Autodesk Fusion 360 part; units mm, degrees
note: some values were not read from the file. Set by a fixed rule: which sketch regions a step uses.
(part 8 of 59)
  spline S40 degree 5 poles (-13.0527, 40.6181) (-13.0525, 40.6154) (-13.0521, 40.61) (-13.0515, 40.6019) (-13.0506, 40.5911) (-13.0495, 40.5777) (-13.0484, 40.5644) (-13.0473, 40.551) (-13.0462, 40.5377) (-13.0451, 40.5244) (-13.0439, 40.5112) (-13.0427, 40.4979) (-13.0415, 40.4848) (-13.0404, 40.4716) (-13.0391, 40.4585) (-13.0379, 40.4454) (-13.0367, 40.4323) (-13.0354, 40.4193) (-13.0342, 40.4063) (-13.0329, 40.3934) (-13.0316, 40.3805) (-13.0303, 40.3676) (-13.029, 40.3547) (-13.0276, 40.3419) (-13.0263, 40.3291) (-13.0249, 40.3164) (-13.0236, 40.3037) (-13.0222, 40.291) (-13.0208, 40.2784) (-13.0194, 40.2658) (-13.018, 40.2532) (-13.0165, 40.2406) (-13.0151, 40.2281) (-13.0136, 40.2157) (-13.0122, 40.2032) (-13.0107, 40.1908) (-13.0092, 40.1785) (-13.0077, 40.1661) (-13.0062, 40.1539) (-13.0047, 40.1416) (-13.0031, 40.1294) (-13.0016, 40.1172) (-13, 40.105) (-12.9984, 40.0929) (-12.9968, 40.0809) (-12.9952, 40.0688) (-12.9936, 40.0568) (-12.992, 40.0449) (-12.9904, 40.0329) (-12.9887, 40.021) (-12.9871, 40.0092) (-12.9854, 39.9974) (-12.9838, 39.9856) (-12.9821, 39.9738) (-12.9804, 39.9621) (-12.9787, 39.9505) (-12.977, 39.9388) (-12.9752, 39.9273) (-12.9735, 39.9157) (-12.9718, 39.9042) (-12.97, 39.8927) (-12.9682, 39.8813) (-12.9665, 39.8699) (-12.9647, 39.8585) (-12.9629, 39.8472) (-12.9611, 39.8359) (-12.9593, 39.8247) (-12.9574, 39.8135) (-12.9556, 39.8023) (-12.9538, 39.7912) (-12.9519, 39.7801) (-12.9501, 39.7691) (-12.9482, 39.7581) (-12.9463, 39.7471) (-12.9445, 39.7362) (-12.9426, 39.7253) (-12.9407, 39.7145) (-12.9388, 39.7037) (-12.9368, 39.6929) (-12.9349, 39.6822) (-12.933, 39.6715) (-12.9311, 39.6609) (-12.9291, 39.6503) (-12.9272, 39.6397) (-12.9252, 39.6292) (-12.9232, 39.6188) (-12.9213, 39.6083) (-12.9193, 39.5979) (-12.9173, 39.5876) (-12.9153, 39.5773) (-12.9133, 39.5671) (-12.9113, 39.5568) (-12.9093, 39.5467) (-12.9072, 39.5365) (-12.9052, 39.5265) (-12.9032, 39.5164) (-12.9011, 39.5064) (-12.8991, 39.4965) (-12.8971, 39.4866) (-12.895, 39.4767) (-12.8929, 39.4669) (-12.8909, 39.4571) (-12.8888, 39.4474) (-12.8867, 39.4377) (-12.8847, 39.4281) (-12.8826, 39.4185) (-12.8805, 39.4089) (-12.8784, 39.3994) (-12.8763, 39.39) (-12.8742, 39.3806) (-12.8721, 39.3712) (-12.87, 39.3619) (-12.8679, 39.3526) (-12.8658, 39.3434) (-12.8636, 39.3342) (-12.8615, 39.3251) (-12.8594, 39.316) (-12.8573, 39.3069) (-12.8551, 39.298) (-12.853, 39.289) (-12.8509, 39.2801) (-12.8487, 39.2713) (-12.8466, 39.2625) (-12.8445, 39.2537) (-12.8423, 39.2451) (-12.8402, 39.2364) (-12.838, 39.2278) (-12.8359, 39.2193) (-12.8337, 39.2108) (-12.8316, 39.2023) (-12.8294, 39.1939) (-12.8273, 39.1856) (-12.8251, 39.1773) (-12.823, 39.169) (-12.8208, 39.1608) (-12.8187, 39.1527) (-12.8166, 39.1446) (-12.8144, 39.1365) (-12.8123, 39.1286) (-12.8101, 39.1206) (-12.808, 39.1127) (-12.8058, 39.1049) (-12.8037, 39.0971) (-12.8016, 39.0894) (-12.7994, 39.0817) (-12.7973, 39.0741) (-12.7952, 39.0665) (-12.793, 39.059) (-12.7909, 39.0516) (-12.7888, 39.0442) (-12.7867, 39.0368) (-12.7845, 39.0296) (-12.7824, 39.0223) (-12.7803, 39.0151) (-12.7782, 39.008) (-12.7761, 39.0009) (-12.774, 38.9939) (-12.772, 38.987) (-12.7699, 38.9801) (-12.7678, 38.9733) (-12.7657, 38.9665) (-12.7637, 38.9598) (-12.7616, 38.9531) (-12.7596, 38.9465) (-12.7575, 38.9399) (-12.7555, 38.9335) (-12.7534, 38.927) (-12.7514, 38.9207) (-12.7494, 38.9144) (-12.7474, 38.9081) (-12.7454, 38.9019) (-12.7434, 38.8958) (-12.7414, 38.8897) (-12.7395, 38.8837) (-12.7375, 38.8778) (-12.7356, 38.8719) (-12.7336, 38.8661) (-12.7317, 38.8604) (-12.7298, 38.8547) (-12.7279, 38.8491) (-12.726, 38.8435) (-12.7241, 38.838) (-12.7222, 38.8326) (-12.7204, 38.8273) (-12.7185, 38.822) (-12.7167, 38.8167) (-12.7149, 38.8116) (-12.7131, 38.8065) (-12.7113, 38.8015) (-12.7095, 38.7965) (-12.7077, 38.7916) (-12.706, 38.7868) (-12.7043, 38.782) (-12.7026, 38.7774) (-12.7009, 38.7728) (-12.6992, 38.7682) (-12.6975, 38.7638) (-12.6959, 38.7594) (-12.6943, 38.755) (-12.6927, 38.7508) (-12.6911, 38.7466) (-12.6895, 38.7425) (-12.688, 38.7385) (-12.6864, 38.7345) (-12.6849, 38.7307) (-12.6834, 38.7269) (-12.682, 38.7231) (-12.6806, 38.7195) (-12.6791, 38.7159) (-12.6778, 38.7124) (-12.6764, 38.709) (-12.675, 38.7057) (-12.6737, 38.7024) (-12.6724, 38.6993) (-12.6712, 38.6962) (-12.6699, 38.6932) (-12.6687, 38.6903) (-12.6676, 38.6874) (-12.6664, 38.6847) (-12.6653, 38.682) (-12.6642, 38.6794) (-12.6631, 38.6769) (-12.6621, 38.6745) (-12.6611, 38.6722) (-12.6602, 38.67) (-12.6592, 38.6678) (-12.6583, 38.6658) (-12.6575, 38.6638) (-12.6567, 38.6619) (-12.6559, 38.6602) (-12.6551, 38.6585) (-12.6544, 38.6569) (-12.6538, 38.6554) (-12.6531, 38.654) (-12.6526, 38.6527) (-12.652, 38.6515) (-12.6515, 38.6504) (-12.651, 38.6495) (-12.6506, 38.6486) (-12.6503, 38.6478) (-12.65, 38.6471) (-12.6497, 38.6467) (-12.6496, 38.6464) (-12.6495, 38.6462) (-12.6495, 38.6461) knots -1 -1 -1 -1 -1 -1 -0.99583333 -0.99166667 -0.9875 -0.98333333 -0.97916667 -0.975 -0.97083333 -0.96666667 -0.9625 -0.95833333 -0.95416667 -0.95 -0.94583333 -0.94166667 -0.9375 -0.93333333 -0.92916667 -0.925 -0.92083333 -0.91666667 -0.9125 -0.90833333 -0.90416667 -0.9 -0.89583333 -0.89166667 -0.8875 -0.88333333 -0.87916667 -0.875 -0.87083333 -0.86666667 -0.8625 -0.85833333 -0.85416667 -0.85 -0.84583333 -0.84166667 -0.8375 -0.83333333 -0.82916667 -0.825 -0.82083333 -0.81666667 -0.8125 -0.80833333 -0.80416667 -0.8 -0.79583333 -0.79166667 -0.7875 -0.78333333 -0.77916667 -0.775 -0.77083333 -0.76666667 -0.7625 -0.75833333 -0.75416667 -0.75 -0.74583333 -0.74166667 -0.7375 -0.73333333 -0.72916667 -0.725 -0.72083333 -0.71666667 -0.7125 -0.70833333 -0.70416667 -0.7 -0.69583333 -0.69166667 -0.6875 -0.68333333 -0.67916667 -0.675 -0.67083333 -0.66666667 -0.6625 -0.65833333 -0.65416667 -0.65 -0.64583333 -0.64166667 -0.6375 -0.63333333 -0.62916667 -0.625 -0.62083333 -0.61666667 -0.6125 -0.60833333 -0.60416667 -0.6 -0.59583333 -0.59166667 -0.5875 -0.58333333 -0.57916667 -0.575 -0.57083333 -0.56666667 -0.5625 -0.55833333 -0.55416667 -0.55 -0.54583333 -0.54166667 -0.5375 -0.53333333 -0.52916667 -0.525 -0.52083333 -0.51666667 -0.5125 -0.50833333 -0.50416667 -0.5 -0.49583333 -0.49166667 -0.4875 -0.48333333 -0.47916667 -0.475 -0.47083333 -0.46666667 -0.4625 -0.45833333 -0.45416667 -0.45 -0.44583333 -0.44166667 -0.4375 -0.43333333 -0.42916667 -0.425 -0.42083333 -0.41666667 -0.4125 -0.40833333 -0.40416667 -0.4 -0.39583333 -0.39166667 -0.3875 -0.38333333 -0.37916667 -0.375 -0.37083333 -0.36666667 -0.3625 -0.35833333 -0.35416667 -0.35 -0.34583333 -0.34166667 -0.3375 -0.33333333 -0.32916667 -0.325 -0.32083333 -0.31666667 -0.3125 -0.30833333 -0.30416667 -0.3 -0.29583333 -0.29166667 -0.2875 -0.28333333 -0.27916667 -0.275 -0.27083333 -0.26666667 -0.2625 -0.25833333 -0.25416667 -0.25 -0.24583333 -0.24166667 -0.2375 -0.23333333 -0.22916667 -0.225 -0.22083333 -0.21666667 -0.2125 -0.20833333 -0.20416667 -0.2 -0.19583333 -0.19166667 -0.1875 -0.18333333 -0.17916667 -0.175 -0.17083333 -0.16666667 -0.1625 -0.15833333 -0.15416667 -0.15 -0.14583333 -0.14166667 -0.1375 -0.13333333 -0.12916667 -0.125 -0.12083333 -0.11666667 -0.1125 -0.10833333 -0.10416667 -0.1 -0.09583333 -0.09166667 -0.0875 -0.08333333 -0.07916667 -0.075 -0.07083333 -0.06666667 -0.0625 -0.05833333 -0.05416667 -0.05 -0.04583333 -0.04166667 -0.0375 -0.03333333 -0.02916667 -0.025 -0.02083333 -0.01666667 -0.0125 -0.00833333 -0.00416667 0 0 0 0 0 0
  spline S41 degree 5 poles (-20.3781, -10.8609) (-20.3757, -10.8596) (-20.371, -10.8571) (-20.3639, -10.8532) (-20.3544, -10.848) (-20.3426, -10.8416) (-20.3308, -10.8351) (-20.319, -10.8287) (-20.3073, -10.8222) (-20.2957, -10.8158) (-20.284, -10.8094) (-20.2724, -10.8029) (-20.2609, -10.7965) (-20.2493, -10.79) (-20.2379, -10.7836) (-20.2264, -10.7771) (-20.215, -10.7707) (-20.2036, -10.7643) (-20.1922, -10.7578) (-20.1809, -10.7514) (-20.1697, -10.745) (-20.1584, -10.7385) (-20.1472, -10.7321) (-20.136, -10.7257) (-20.1249, -10.7193) (-20.1138, -10.7128) (-20.1028, -10.7064) (-20.0917, -10.7) (-20.0808, -10.6936) (-20.0698, -10.6872) (-20.0589, -10.6807) (-20.048, -10.6743) (-20.0372, -10.6679) (-20.0264, -10.6615) (-20.0156, -10.6551) (-20.0049, -10.6487) (-19.9942, -10.6423) (-19.9836, -10.636) (-19.973, -10.6296) (-19.9624, -10.6232) (-19.9518, -10.6168) (-19.9413, -10.6104) (-19.9309, -10.6041) (-19.9205, -10.5977) (-19.9101, -10.5914) (-19.8997, -10.585) (-19.8894, -10.5786) (-19.8791, -10.5723) (-19.8689, -10.566) (-19.8587, -10.5596) (-19.8486, -10.5533) (-19.8384, -10.547) (-19.8284, -10.5406) (-19.8183, -10.5343) (-19.8083, -10.528) (-19.7984, -10.5217) (-19.7884, -10.5154) (-19.7785, -10.5091) (-19.7687, -10.5029) (-19.7589, -10.4966) (-19.7491, -10.4903) (-19.7394, -10.484) (-19.7297, -10.4778) (-19.72, -10.4715) (-19.7104, -10.4653) (-19.7009, -10.4591) (-19.6913, -10.4528) (-19.6818, -10.4466) (-19.6724, -10.4404) (-19.663, -10.4342) (-19.6536, -10.428) (-19.6443, -10.4218) (-19.635, -10.4156) (-19.6257, -10.4095) (-19.6165, -10.4033) (-19.6073, -10.3971) (-19.5982, -10.391) (-19.5891, -10.3849) (-19.5801, -10.3787) (-19.5711, -10.3726) (-19.5621, -10.3665) (-19.5532, -10.3604) (-19.5443, -10.3543) (-19.5354, -10.3483) (-19.5266, -10.3422) (-19.5179, -10.3361) (-19.5091, -10.3301) (-19.5005, -10.3241) (-19.4918, -10.318) (-19.4832, -10.312) (-19.4747, -10.306) (-19.4662, -10.3) (-19.4577, -10.2941) (-19.4493, -10.2881) (-19.4409, -10.2822) (-19.4325, -10.2762) (-19.4242, -10.2703) (-19.416, -10.2644) (-19.4078, -10.2585) (-19.3996, -10.2526) (-19.3914, -10.2467) (-19.3834, -10.2408) (-19.3753, -10.235) (-19.3673, -10.2292) (-19.3593, -10.2233) (-19.3514, -10.2175) (-19.3436, -10.2118) (-19.3357, -10.206) (-19.3279, -10.2002) (-19.3202, -10.1945) (-19.3125, -10.1887) (-19.3048, -10.183) (-19.2972, -10.1773) (-19.2897, -10.1716) (-19.2821, -10.166) (-19.2747, -10.1603) (-19.2672, -10.1547) (-19.2598, -10.1491) (-19.2525, -10.1435) (-19.2452, -10.1379) (-19.2379, -10.1323) (-19.2307, -10.1268) (-19.2236, -10.1212) (-19.2165, -10.1157) (-19.2094, -10.1102) (-19.2024, -10.1048) (-19.1954, -10.0993) (-19.1884, -10.0939) (-19.1815, -10.0884) (-19.1747, -10.083) (-19.1679, -10.0777) (-19.1611, -10.0723) (-19.1544, -10.067) (-19.1478, -10.0617) (-19.1412, -10.0564) (-19.1346, -10.0511) (-19.1281, -10.0458) (-19.1216, -10.0406) (-19.1152, -10.0354) (-19.1088, -10.0302) (-19.1025, -10.025) (-19.0962, -10.0199) (-19.09, -10.0148) (-19.0838, -10.0097) (-19.0776, -10.0046) (-19.0715, -9.9996) (-19.0655, -9.9945) (-19.0595, -9.9895) (-19.0536, -9.9846) (-19.0477, -9.9796) (-19.0418, -9.9747) (-19.036, -9.9698) (-19.0303, -9.9649) (-19.0246, -9.9601) (-19.0189, -9.9553) (-19.0133, -9.9505) (-19.0077, -9.9457) (-19.0022, -9.941) (-18.9968, -9.9363) (-18.9914, -9.9316) (-18.986, -9.927) (-18.9807, -9.9223) (-18.9755, -9.9177) (-18.9703, -9.9132) (-18.9651, -9.9087) (-18.96, -9.9042) (-18.955, -9.8997) (-18.95, -9.8953) (-18.9451, -9.8909) (-18.9402, -9.8865) (-18.9353, -9.8821) (-18.9306, -9.8778) (-18.9258, -9.8736) (-18.9211, -9.8693) (-18.9165, -9.8651) (-18.9119, -9.8609) (-18.9074, -9.8568) (-18.903, -9.8527) (-18.8986, -9.8486) (-18.8942, -9.8446) (-18.8899, -9.8406) (-18.8856, -9.8367) (-18.8814, -9.8328) (-18.8773, -9.8289) (-18.8732, -9.825) (-18.8692, -9.8212) (-18.8652, -9.8175) (-18.8613, -9.8138) (-18.8574, -9.8101) (-18.8536, -9.8065) (-18.8499, -9.8029) (-18.8462, -9.7993) (-18.8426, -9.7958) (-18.839, -9.7923) (-18.8355, -9.7889) (-18.832, -9.7855) (-18.8286, -9.7822) (-18.8252, -9.7789) (-18.822, -9.7757) (-18.8187, -9.7725) (-18.8156, -9.7693) (-18.8124, -9.7662) (-18.8094, -9.7632) (-18.8064, -9.7602) (-18.8035, -9.7572) (-18.8006, -9.7543) (-18.7978, -9.7515) (-18.7951, -9.7487) (-18.7924, -9.7459) (-18.7897, -9.7433) (-18.7872, -9.7406) (-18.7847, -9.738) (-18.7823, -9.7355) (-18.7799, -9.7331) (-18.7776, -9.7307) (-18.7753, -9.7283) (-18.7732, -9.726) (-18.771, -9.7238) (-18.769, -9.7216) (-18.767, -9.7195) (-18.7651, -9.7175) (-18.7632, -9.7155) (-18.7615, -9.7136) (-18.7597, -9.7117) (-18.7581, -9.7099) (-18.7565, -9.7082) (-18.755, -9.7066) (-18.7536, -9.705) (-18.7522, -9.7035) (-18.7509, -9.702) (-18.7497, -9.7007) (-18.7485, -9.6994) (-18.7474, -9.6982) (-18.7464, -9.697) (-18.7455, -9.696) (-18.7446, -9.695) (-18.7438, -9.6941) (-18.7431, -9.6933) (-18.7424, -9.6925) (-18.7419, -9.6919) (-18.7414, -9.6913) (-18.741, -9.6909) (-18.7408, -9.6907) (-18.7407, -9.6905) (-18.7406, -9.6904) knots -1 -1 -1 -1 -1 -1 -0.99583333 -0.99166667 -0.9875 -0.98333333 -0.97916667 -0.975 -0.97083333 -0.96666667 -0.9625 -0.95833333 -0.95416667 -0.95 -0.94583333 -0.94166667 -0.9375 -0.93333333 -0.92916667 -0.925 -0.92083333 -0.91666667 -0.9125 -0.90833333 -0.90416667 -0.9 -0.89583333 -0.89166667 -0.8875 -0.88333333 -0.87916667 -0.875 -0.87083333 -0.86666667 -0.8625 -0.85833333 -0.85416667 -0.85 -0.84583333 -0.84166667 -0.8375 -0.83333333 -0.82916667 -0.825 -0.82083333 -0.81666667 -0.8125 -0.80833333 -0.80416667 -0.8 -0.79583333 -0.79166667 -0.7875 -0.78333333 -0.77916667 -0.775 -0.77083333 -0.76666667 -0.7625 -0.75833333 -0.75416667 -0.75 -0.74583333 -0.74166667 -0.7375 -0.73333333 -0.72916667 -0.725 -0.72083333 -0.71666667 -0.7125 -0.70833333 -0.70416667 -0.7 -0.69583333 -0.69166667 -0.6875 -0.68333333 -0.67916667 -0.675 -0.67083333 -0.66666667 -0.6625 -0.65833333 -0.65416667 -0.65 -0.64583333 -0.64166667 -0.6375 -0.63333333 -0.62916667 -0.625 -0.62083333 -0.61666667 -0.6125 -0.60833333 -0.60416667 -0.6 -0.59583333 -0.59166667 -0.5875 -0.58333333 -0.57916667 -0.575 -0.57083333 -0.56666667 -0.5625 -0.55833333 -0.55416667 -0.55 -0.54583333 -0.54166667 -0.5375 -0.53333333 -0.52916667 -0.525 -0.52083333 -0.51666667 -0.5125 -0.50833333 -0.50416667 -0.5 -0.49583333 -0.49166667 -0.4875 -0.48333333 -0.47916667 -0.475 -0.47083333 -0.46666667 -0.4625 -0.45833333 -0.45416667 -0.45 -0.44583333 -0.44166667 -0.4375 -0.43333333 -0.42916667 -0.425 -0.42083333 -0.41666667 -0.4125 -0.40833333 -0.40416667 -0.4 -0.39583333 -0.39166667 -0.3875 -0.38333333 -0.37916667 -0.375 -0.37083333 -0.36666667 -0.3625 -0.35833333 -0.35416667 -0.35 -0.34583333 -0.34166667 -0.3375 -0.33333333 -0.32916667 -0.325 -0.32083333 -0.31666667 -0.3125 -0.30833333 -0.30416667 -0.3 -0.29583333 -0.29166667 -0.2875 -0.28333333 -0.27916667 -0.275 -0.27083333 -0.26666667 -0.2625 -0.25833333 -0.25416667 -0.25 -0.24583333 -0.24166667 -0.2375 -0.23333333 -0.22916667 -0.225 -0.22083333 -0.21666667 -0.2125 -0.20833333 -0.20416667 -0.2 -0.19583333 -0.19166667 -0.1875 -0.18333333 -0.17916667 -0.175 -0.17083333 -0.16666667 -0.1625 -0.15833333 -0.15416667 -0.15 -0.14583333 -0.14166667 -0.1375 -0.13333333 -0.12916667 -0.125 -0.12083333 -0.11666667 -0.1125 -0.10833333 -0.10416667 -0.1 -0.09583333 -0.09166667 -0.0875 -0.08333333 -0.07916667 -0.075 -0.07083333 -0.06666667 -0.0625 -0.05833333 -0.05416667 -0.05 -0.04583333 -0.04166667 -0.0375 -0.03333333 -0.02916667 -0.025 -0.02083333 -0.01666667 -0.0125 -0.00833333 -0.00416667 0 0 0 0 0 0
  spline S42 degree 5 poles (-15.9204, 39.0997) (-15.9199, 39.097) (-15.9189, 39.0917) (-15.9174, 39.0837) (-15.9154, 39.0731) (-15.913, 39.0599) (-15.9105, 39.0467) (-15.908, 39.0335) (-15.9055, 39.0204) (-15.9029, 39.0073) (-15.9004, 38.9943) (-15.8979, 38.9812) (-15.8953, 38.9682) (-15.8927, 38.9553) (-15.8902, 38.9424) (-15.8876, 38.9295) (-15.885, 38.9166) (-15.8824, 38.9038) (-15.8798, 38.891) (-15.8771, 38.8783) (-15.8745, 38.8656) (-15.8719, 38.8529) (-15.8692, 38.8403) (-15.8666, 38.8276) (-15.8639, 38.8151) (-15.8612, 38.8025) (-15.8585, 38.79) (-15.8558, 38.7776) (-15.8531, 38.7651) (-15.8504, 38.7528) (-15.8477, 38.7404) (-15.8449, 38.7281) (-15.8422, 38.7158) (-15.8394, 38.7035) (-15.8367, 38.6913) (-15.8339, 38.6792) (-15.8311, 38.667) (-15.8283, 38.6549) (-15.8255, 38.6428) (-15.8227, 38.6308) (-15.8199, 38.6188) (-15.8171, 38.6069) (-15.8143, 38.595) (-15.8115, 38.5831) (-15.8086, 38.5712) (-15.8058, 38.5594) (-15.8029, 38.5477) (-15.8001, 38.5359) (-15.7972, 38.5242) (-15.7943, 38.5126) (-15.7914, 38.501) (-15.7886, 38.4894) (-15.7857, 38.4778) (-15.7828, 38.4663) (-15.7798, 38.4549) (-15.7769, 38.4435) (-15.774, 38.4321) (-15.7711, 38.4207) (-15.7682, 38.4094) (-15.7652, 38.3982) (-15.7623, 38.3869) (-15.7593, 38.3757) (-15.7564, 38.3646) (-15.7534, 38.3535) (-15.7504, 38.3424) (-15.7475, 38.3314) (-15.7445, 38.3204) (-15.7415, 38.3094) (-15.7385, 38.2985) (-15.7355, 38.2877) (-15.7325, 38.2768) (-15.7295, 38.266) (-15.7265, 38.2553) (-15.7235, 38.2446) (-15.7205, 38.2339) (-15.7175, 38.2233) (-15.7145, 38.2127) (-15.7114, 38.2022) (-15.7084, 38.1917) (-15.7054, 38.1812) (-15.7023, 38.1708) (-15.6993, 38.1604) (-15.6963, 38.1501) (-15.6932, 38.1398) (-15.6902, 38.1296) (-15.6871, 38.1194) (-15.6841, 38.1092) (-15.681, 38.0991) (-15.6779, 38.089) (-15.6749, 38.079) (-15.6718, 38.069) (-15.6688, 38.059) (-15.6657, 38.0491) (-15.6626, 38.0393) (-15.6596, 38.0294) (-15.6565, 38.0197) (-15.6534, 38.0099) (-15.6503, 38.0003) (-15.6473, 37.9906) (-15.6442, 37.981) (-15.6411, 37.9715) (-15.638, 37.962) (-15.635, 37.9525) (-15.6319, 37.9431) (-15.6288, 37.9337) (-15.6257, 37.9244) (-15.6227, 37.9151) (-15.6196, 37.9059) (-15.6165, 37.8967) (-15.6134, 37.8876) (-15.6104, 37.8785) (-15.6073, 37.8694) (-15.6042, 37.8604) (-15.6012, 37.8515) (-15.5981, 37.8426) (-15.595, 37.8337) (-15.592, 37.8249) (-15.5889, 37.8161) (-15.5859, 37.8074) (-15.5828, 37.7988) (-15.5798, 37.7901) (-15.5767, 37.7816) (-15.5737, 37.7731) (-15.5706, 37.7646) (-15.5676, 37.7562) (-15.5645, 37.7478) (-15.5615, 37.7394) (-15.5585, 37.7312) (-15.5555, 37.7229) (-15.5524, 37.7148) (-15.5494, 37.7066) (-15.5464, 37.6986) (-15.5434, 37.6905) (-15.5404, 37.6826) (-15.5374, 37.6746) (-15.5344, 37.6668) (-15.5315, 37.6589) (-15.5285, 37.6512) (-15.5255, 37.6434) (-15.5226, 37.6358) (-15.5196, 37.6282) (-15.5166, 37.6206) (-15.5137, 37.6131) (-15.5108, 37.6056) (-15.5078, 37.5982) (-15.5049, 37.5909) (-15.502, 37.5836) (-15.4991, 37.5763) (-15.4962, 37.5691) (-15.4933, 37.562) (-15.4905, 37.5549) (-15.4876, 37.5479) (-15.4848, 37.5409) (-15.4819, 37.534) (-15.4791, 37.5271) (-15.4762, 37.5203) (-15.4734, 37.5136) (-15.4706, 37.5069) (-15.4678, 37.5002) (-15.4651, 37.4936) (-15.4623, 37.4871) (-15.4595, 37.4806) (-15.4568, 37.4742) (-15.4541, 37.4679) (-15.4514, 37.4616) (-15.4486, 37.4553) (-15.446, 37.4492) (-15.4433, 37.443) (-15.4406, 37.437) (-15.438, 37.431) (-15.4353, 37.425) (-15.4327, 37.4192) (-15.4301, 37.4133) (-15.4275, 37.4076) (-15.425, 37.4019) (-15.4224, 37.3962) (-15.4199, 37.3907) (-15.4174, 37.3852) (-15.4149, 37.3797) (-15.4124, 37.3743) (-15.4099, 37.369) (-15.4075, 37.3637) (-15.405, 37.3585) (-15.4026, 37.3534) (-15.4002, 37.3483) (-15.3979, 37.3433) (-15.3955, 37.3384) (-15.3932, 37.3335) (-15.3909, 37.3287) (-15.3886, 37.3239) (-15.3863, 37.3193) (-15.3841, 37.3147) (-15.3819, 37.3101) (-15.3797, 37.3056) (-15.3775, 37.3012) (-15.3754, 37.2969) (-15.3733, 37.2926) (-15.3712, 37.2884) (-15.3691, 37.2843) (-15.3671, 37.2802) (-15.3651, 37.2763) (-15.3631, 37.2723) (-15.3611, 37.2685) (-15.3592, 37.2647) (-15.3573, 37.261) (-15.3554, 37.2574) (-15.3536, 37.2539) (-15.3518, 37.2504) (-15.35, 37.247) (-15.3482, 37.2437) (-15.3465, 37.2404) (-15.3449, 37.2372) (-15.3432, 37.2341) (-15.3416, 37.2311) (-15.34, 37.2282) (-15.3385, 37.2253) (-15.337, 37.2225) (-15.3355, 37.2198) (-15.3341, 37.2172) (-15.3327, 37.2147) (-15.3313, 37.2122) (-15.33, 37.2099) (-15.3287, 37.2076) (-15.3275, 37.2054) (-15.3263, 37.2033) (-15.3252, 37.2012) (-15.3241, 37.1993) (-15.323, 37.1974) (-15.322, 37.1956) (-15.321, 37.194) (-15.3201, 37.1924) (-15.3193, 37.1909) (-15.3184, 37.1895) (-15.3177, 37.1881) (-15.3169, 37.1869) (-15.3163, 37.1858) (-15.3157, 37.1848) (-15.3151, 37.1838) (-15.3146, 37.183) (-15.3142, 37.1822) (-15.3138, 37.1816) (-15.3135, 37.1812) (-15.3133, 37.1809) (-15.3132, 37.1807) (-15.3132, 37.1806) knots -1 -1 -1 -1 -1 -1 -0.99583333 -0.99166667 -0.9875 -0.98333333 -0.97916667 -0.975 -0.97083333 -0.96666667 -0.9625 -0.95833333 -0.95416667 -0.95 -0.94583333 -0.94166667 -0.9375 -0.93333333 -0.92916667 -0.925 -0.92083333 -0.91666667 -0.9125 -0.90833333 -0.90416667 -0.9 -0.89583333 -0.89166667 -0.8875 -0.88333333 -0.87916667 -0.875 -0.87083333 -0.86666667 -0.8625 -0.85833333 -0.85416667 -0.85 -0.84583333 -0.84166667 -0.8375 -0.83333333 -0.82916667 -0.825 -0.82083333 -0.81666667 -0.8125 -0.80833333 -0.80416667 -0.8 -0.79583333 -0.79166667 -0.7875 -0.78333333 -0.77916667 -0.775 -0.77083333 -0.76666667 -0.7625 -0.75833333 -0.75416667 -0.75 -0.74583333 -0.74166667 -0.7375 -0.73333333 -0.72916667 -0.725 -0.72083333 -0.71666667 -0.7125 -0.70833333 -0.70416667 -0.7 -0.69583333 -0.69166667 -0.6875 -0.68333333 -0.67916667 -0.675 -0.67083333 -0.66666667 -0.6625 -0.65833333 -0.65416667 -0.65 -0.64583333 -0.64166667 -0.6375 -0.63333333 -0.62916667 -0.625 -0.62083333 -0.61666667 -0.6125 -0.60833333 -0.60416667 -0.6 -0.59583333 -0.59166667 -0.5875 -0.58333333 -0.57916667 -0.575 -0.57083333 -0.56666667 -0.5625 -0.55833333 -0.55416667 -0.55 -0.54583333 -0.54166667 -0.5375 -0.53333333 -0.52916667 -0.525 -0.52083333 -0.51666667 -0.5125 -0.50833333 -0.50416667 -0.5 -0.49583333 -0.49166667 -0.4875 -0.48333333 -0.47916667 -0.475 -0.47083333 -0.46666667 -0.4625 -0.45833333 -0.45416667 -0.45 -0.44583333 -0.44166667 -0.4375 -0.43333333 -0.42916667 -0.425 -0.42083333 -0.41666667 -0.4125 -0.40833333 -0.40416667 -0.4 -0.39583333 -0.39166667 -0.3875 -0.38333333 -0.37916667 -0.375 -0.37083333 -0.36666667 -0.3625 -0.35833333 -0.35416667 -0.35 -0.34583333 -0.34166667 -0.3375 -0.33333333 -0.32916667 -0.325 -0.32083333 -0.31666667 -0.3125 -0.30833333 -0.30416667 -0.3 -0.29583333 -0.29166667 -0.2875 -0.28333333 -0.27916667 -0.275 -0.27083333 -0.26666667 -0.2625 -0.25833333 -0.25416667 -0.25 -0.24583333 -0.24166667 -0.2375 -0.23333333 -0.22916667 -0.225 -0.22083333 -0.21666667 -0.2125 -0.20833333 -0.20416667 -0.2 -0.19583333 -0.19166667 -0.1875 -0.18333333 -0.17916667 -0.175 -0.17083333 -0.16666667 -0.1625 -0.15833333 -0.15416667 -0.15 -0.14583333 -0.14166667 -0.1375 -0.13333333 -0.12916667 -0.125 -0.12083333 -0.11666667 -0.1125 -0.10833333 -0.10416667 -0.1 -0.09583333 -0.09166667 -0.0875 -0.08333333 -0.07916667 -0.075 -0.07083333 -0.06666667 -0.0625 -0.05833333 -0.05416667 -0.05 -0.04583333 -0.04166667 -0.0375 -0.03333333 -0.02916667 -0.025 -0.02083333 -0.01666667 -0.0125 -0.00833333 -0.00416667 0 0 0 0 0 0
  line L102 (-17.8091, 35.4448) -> (-17.8086, 35.4441)
  line L103 (-18.7401, 34.6898) -> (-18.7406, 34.6904)
  line L104 (-20.1094, 33.4569) -> (-19.9055, 33.2445)
  line L105 (-20.7445, 32.4055) -> (-20.9569, 32.6094)
  line L106 (-16.318, 36.5271) -> (-16.3184, 36.5278)
  line L107 (-5.0824, 40.7972) -> (-5.1345, 41.087)
  arc A51 (-15.1575, 36.9297) -> (-16.1526, 36.2836) centre (0, 12.5) ccw
  line L108 (-5.1345, 41.087) -> (-5.1346, 41.0878)
  arc A52 (-0.9119, 41.2355) -> (-2.0967, 41.1734) centre (0, 12.5) ccw
  line L109 (-15.3128, 37.1799) -> (-15.1575, 36.9297)
  arc A53 (-2.755, 43.3773) -> (-3.7249, 43.2754) centre (0, 12.5) ccw
  line L110 (-18.5501, 34.4649) -> (-18.7401, 34.6898)
  line L111 (-20.11, 33.4575) -> (-20.1094, 33.4569)
  arc A54 (-3.9106, 40.9828) -> (-5.0824, 40.7972) centre (0, 12.5) ccw
  line L112 (-17.8086, 35.4441) -> (-17.6281, 35.2115)
  spline S43 degree 5 poles (-2.1183, 41.4679) (-2.1183, 41.468) (-2.1183, 41.4682) (-2.1183, 41.4685) (-2.1184, 41.469) (-2.1184, 41.4698) (-2.1185, 41.4706) (-2.1186, 41.4716) (-2.1187, 41.4727) (-2.1188, 41.4739) (-2.1189, 41.4752) (-2.1191, 41.4766) (-2.1192, 41.4781) (-2.1194, 41.4798) (-2.1196, 41.4815) (-2.1198, 41.4833) (-2.12, 41.4852) (-2.1202, 41.4873) (-2.1204, 41.4894) (-2.1207, 41.4916) (-2.121, 41.4939) (-2.1212, 41.4963) (-2.1215, 41.4989) (-2.1219, 41.5015) (-2.1222, 41.5041) (-2.1225, 41.5069) (-2.1229, 41.5098) (-2.1233, 41.5128) (-2.1237, 41.5158) (-2.1241, 41.5189) (-2.1245, 41.5222) (-2.125, 41.5255) (-2.1254, 41.5289) (-2.1259, 41.5323) (-2.1264, 41.5359) (-2.127, 41.5395) (-2.1275, 41.5432) (-2.1281, 41.547) (-2.1286, 41.5509) (-2.1292, 41.5549) (-2.1299, 41.5589) (-2.1305, 41.563) (-2.1312, 41.5672) (-2.1318, 41.5714) (-2.1325, 41.5758) (-2.1332, 41.5802) (-2.134, 41.5847) (-2.1347, 41.5892) (-2.1355, 41.5938) (-2.1363, 41.5985) (-2.1371, 41.6033) (-2.138, 41.6081) (-2.1388, 41.6131) (-2.1397, 41.618) (-2.1406, 41.6231) (-2.1415, 41.6282) (-2.1424, 41.6334) (-2.1434, 41.6386) (-2.1444, 41.6439) (-2.1454, 41.6493) (-2.1464, 41.6547) (-2.1475, 41.6602) (-2.1485, 41.6658) (-2.1496, 41.6714) (-2.1507, 41.6771) (-2.1519, 41.6829) (-2.153, 41.6887) (-2.1542, 41.6946) (-2.1554, 41.7005) (-2.1567, 41.7065) (-2.1579, 41.7126) (-2.1592, 41.7187) (-2.1605, 41.7249) (-2.1618, 41.7311) (-2.1631, 41.7374) (-2.1645, 41.7438) (-2.1659, 41.7502) (-2.1673, 41.7567) (-2.1687, 41.7632) (-2.1702, 41.7698) (-2.1716, 41.7764) (-2.1731, 41.7831) (-2.1747, 41.7899) (-2.1762, 41.7967) (-2.1778, 41.8035) (-2.1794, 41.8104) (-2.181, 41.8174) (-2.1827, 41.8244) (-2.1843, 41.8314) (-2.186, 41.8386) (-2.1877, 41.8457) (-2.1895, 41.8529) (-2.1912, 41.8602) (-2.193, 41.8675) (-2.1948, 41.8749) (-2.1967, 41.8823) (-2.1985, 41.8898) (-2.2004, 41.8973) (-2.2023, 41.9049) (-2.2043, 41.9125) (-2.2062, 41.9202) (-2.2082, 41.9279) (-2.2102, 41.9356) (-2.2123, 41.9434) (-2.2143, 41.9513) (-2.2164, 41.9592) (-2.2185, 41.9671) (-2.2207, 41.9751) (-2.2228, 41.9832) (-2.225, 41.9912) (-2.2272, 41.9994) (-2.2295, 42.0075) (-2.2317, 42.0158) (-2.234, 42.024) (-2.2363, 42.0323) (-2.2387, 42.0407) (-2.241, 42.0491) (-2.2434, 42.0575) (-2.2458, 42.066) (-2.2483, 42.0745) (-2.2508, 42.083) (-2.2533, 42.0917) (-2.2558, 42.1003) (-2.2583, 42.109) (-2.2609, 42.1177) (-2.2635, 42.1265) (-2.2661, 42.1353) (-2.2688, 42.1441) (-2.2714, 42.153) (-2.2741, 42.1619) (-2.2769, 42.1709) (-2.2796, 42.1799) (-2.2824, 42.189) (-2.2852, 42.1981) (-2.288, 42.2072) (-2.2909, 42.2163) (-2.2938, 42.2255) (-2.2967, 42.2348) (-2.2996, 42.2441) (-2.3026, 42.2534) (-2.3056, 42.2627) (-2.3086, 42.2721) (-2.3117, 42.2815) (-2.3147, 42.291) (-2.3178, 42.3005) (-2.321, 42.31) (-2.3241, 42.3196) (-2.3273, 42.3292) (-2.3305, 42.3388) (-2.3337, 42.3485) (-2.337, 42.3582) (-2.3403, 42.368) (-2.3436, 42.3777) (-2.3469, 42.3875) (-2.3503, 42.3974) (-2.3537, 42.4073) (-2.3571, 42.4172) (-2.3606, 42.4271) (-2.364, 42.4371) (-2.3675, 42.4471) (-2.3711, 42.4572) (-2.3746, 42.4673) (-2.3782, 42.4774) (-2.3818, 42.4875) (-2.3855, 42.4977) (-2.3891, 42.5079) (-2.3928, 42.5182) (-2.3965, 42.5284) (-2.4003, 42.5388) (-2.4041, 42.5491) (-2.4079, 42.5595) (-2.4117, 42.5699) (-2.4156, 42.5803) (-2.4194, 42.5907) (-2.4234, 42.6012) (-2.4273, 42.6118) (-2.4313, 42.6223) (-2.4353, 42.6329) (-2.4393, 42.6435) (-2.4433, 42.6541) (-2.4474, 42.6648) (-2.4515, 42.6755) (-2.4557, 42.6862) (-2.4598, 42.697) (-2.464, 42.7078) (-2.4682, 42.7186) (-2.4725, 42.7294) (-2.4767, 42.7403) (-2.481, 42.7512) (-2.4854, 42.7621) (-2.4897, 42.7731) (-2.4941, 42.7841) (-2.4985, 42.7951) (-2.503, 42.8061) (-2.5074, 42.8172) (-2.5119, 42.8283) (-2.5165, 42.8394) (-2.521, 42.8506) (-2.5256, 42.8617) (-2.5302, 42.8729) (-2.5348, 42.8841) (-2.5395, 42.8954) (-2.5442, 42.9067) (-2.5489, 42.918) (-2.5537, 42.9293) (-2.5584, 42.9407) (-2.5632, 42.952) (-2.5681, 42.9634) (-2.5729, 42.9749) (-2.5778, 42.9863) (-2.5827, 42.9978) (-2.5877, 43.0093) (-2.5927, 43.0208) (-2.5977, 43.0324) (-2.6027, 43.0439) (-2.6077, 43.0555) (-2.6128, 43.0672) (-2.6179, 43.0788) (-2.6231, 43.0905) (-2.6283, 43.1022) (-2.6335, 43.1139) (-2.6387, 43.1256) (-2.6439, 43.1374) (-2.6492, 43.1492) (-2.6545, 43.161) (-2.6599, 43.1728) (-2.6653, 43.1847) (-2.6707, 43.1966) (-2.6761, 43.2085) (-2.6815, 43.2204) (-2.687, 43.2323) (-2.6925, 43.2443) (-2.6981, 43.2563) (-2.7036, 43.2683) (-2.7092, 43.2803) (-2.7149, 43.2924) (-2.7205, 43.3044) (-2.7262, 43.3165) (-2.7319, 43.3287) (-2.7376, 43.3408) (-2.7434, 43.353) (-2.748, 43.3627) (-2.7515, 43.37) (-2.7539, 43.3749) (-2.755, 43.3773) knots 0 0 0 0 0 0 0.00416667 0.00833333 0.0125 0.01666667 0.02083333 0.025 0.02916667 0.03333333 0.0375 0.04166667 0.04583333 0.05 0.05416667 0.05833333 0.0625 0.06666667 0.07083333 0.075 0.07916667 0.08333333 0.0875 0.09166667 0.09583333 0.1 0.10416667 0.10833333 0.1125 0.11666667 0.12083333 0.125 0.12916667 0.13333333 0.1375 0.14166667 0.14583333 0.15 0.15416667 0.15833333 0.1625 0.16666667 0.17083333 0.175 0.17916667 0.18333333 0.1875 0.19166667 0.19583333 0.2 0.20416667 0.20833333 0.2125 0.21666667 0.22083333 0.225 0.22916667 0.23333333 0.2375 0.24166667 0.24583333 0.25 0.25416667 0.25833333 0.2625 0.26666667 0.27083333 0.275 0.27916667 0.28333333 0.2875 0.29166667 0.29583333 0.3 0.30416667 0.30833333 0.3125 0.31666667 0.32083333 0.325 0.32916667 0.33333333 0.3375 0.34166667 0.34583333 0.35 0.35416667 0.35833333 0.3625 0.36666667 0.37083333 0.375 0.37916667 0.38333333 0.3875 0.39166667 0.39583333 0.4 0.40416667 0.40833333 0.4125 0.41666667 0.42083333 0.425 0.42916667 0.43333333 0.4375 0.44166667 0.44583333 0.45 0.45416667 0.45833333 0.4625 0.46666667 0.47083333 0.475 0.47916667 0.48333333 0.4875 0.49166667 0.49583333 0.5 0.50416667 0.50833333 0.5125 0.51666667 0.52083333 0.525 0.52916667 0.53333333 0.5375 0.54166667 0.54583333 0.55 0.55416667 0.55833333 0.5625 0.56666667 0.57083333 0.575 0.57916667 0.58333333 0.5875 0.59166667 0.59583333 0.6 0.60416667 0.60833333 0.6125 0.61666667 0.62083333 0.625 0.62916667 0.63333333 0.6375 0.64166667 0.64583333 0.65 0.65416667 0.65833333 0.6625 0.66666667 0.67083333 0.675 0.67916667 0.68333333 0.6875 0.69166667 0.69583333 0.7 0.70416667 0.70833333 0.7125 0.71666667 0.72083333 0.725 0.72916667 0.73333333 0.7375 0.74166667 0.74583333 0.75 0.75416667 0.75833333 0.7625 0.76666667 0.77083333 0.775 0.77916667 0.78333333 0.7875 0.79166667 0.79583333 0.8 0.80416667 0.80833333 0.8125 0.81666667 0.82083333 0.825 0.82916667 0.83333333 0.8375 0.84166667 0.84583333 0.85 0.85416667 0.85833333 0.8625 0.86666667 0.87083333 0.875 0.87916667 0.88333333 0.8875 0.89166667 0.89583333 0.9 0.90416667 0.90833333 0.9125 0.91666667 0.92083333 0.925 0.92916667 0.93333333 0.9375 0.94166667 0.94583333 0.95 0.95416667 0.95833333 0.9625 0.96666667 0.97083333 0.975 0.97916667 0.98333333 0.9875 0.99166667 0.99583333 1 1 1 1 1 1
  spline S44 degree 5 poles (-0.4876, 43.4962) (-0.4885, 43.4936) (-0.4903, 43.4885) (-0.493, 43.4809) (-0.4966, 43.4707) (-0.5011, 43.458) (-0.5055, 43.4453) (-0.5099, 43.4327) (-0.5143, 43.4201) (-0.5187, 43.4075) (-0.523, 43.3949) (-0.5273, 43.3823) (-0.5316, 43.3698) (-0.5359, 43.3573) (-0.5401, 43.3448) (-0.5443, 43.3324) (-0.5485, 43.32) (-0.5526, 43.3076) (-0.5568, 43.2952) (-0.5609, 43.2828) (-0.5649, 43.2705) (-0.569, 43.2582) (-0.573, 43.2459) (-0.577, 43.2337) (-0.581, 43.2215) (-0.5849, 43.2093) (-0.5889, 43.1971) (-0.5927, 43.185) (-0.5966, 43.1728) (-0.6005, 43.1607) (-0.6043, 43.1487) (-0.6081, 43.1366) (-0.6118, 43.1246) (-0.6156, 43.1126) (-0.6193, 43.1007) (-0.623, 43.0888) (-0.6267, 43.0769) (-0.6303, 43.065) (-0.6339, 43.0531) (-0.6375, 43.0413) (-0.6411, 43.0295) (-0.6446, 43.0178) (-0.6481, 43.006) (-0.6516, 42.9943) (-0.6551, 42.9827) (-0.6585, 42.971) (-0.6619, 42.9594) (-0.6653, 42.9478) (-0.6687, 42.9362) (-0.672, 42.9247) (-0.6753, 42.9132) (-0.6786, 42.9017) (-0.6819, 42.8903) (-0.6851, 42.8789) (-0.6883, 42.8675) (-0.6915, 42.8562) (-0.6947, 42.8448) (-0.6978, 42.8336) (-0.7009, 42.8223) (-0.704, 42.8111) (-0.7071, 42.7999) (-0.7101, 42.7887) (-0.7131, 42.7776) (-0.7161, 42.7665) (-0.7191, 42.7554) (-0.722, 42.7444) (-0.7249, 42.7334) (-0.7278, 42.7224) (-0.7307, 42.7114) (-0.7335, 42.7005) (-0.7364, 42.6897) (-0.7391, 42.6788) (-0.7419, 42.668) (-0.7447, 42.6572) (-0.7474, 42.6465) (-0.7501, 42.6358) (-0.7528, 42.6251) (-0.7554, 42.6145) (-0.758, 42.6038) (-0.7606, 42.5933) (-0.7632, 42.5827) (-0.7658, 42.5722) (-0.7683, 42.5618) (-0.7708, 42.5513) (-0.7733, 42.5409) (-0.7758, 42.5306) (-0.7782, 42.5202) (-0.7806, 42.5099) (-0.783, 42.4997) (-0.7854, 42.4895) (-0.7877, 42.4793) (-0.79, 42.4691) (-0.7923, 42.459) (-0.7946, 42.449) (-0.7969, 42.4389) (-0.7991, 42.4289) (-0.8013, 42.419) (-0.8035, 42.409) (-0.8056, 42.3992) (-0.8078, 42.3893) (-0.8099, 42.3795) (-0.812, 42.3697) (-0.814, 42.36) (-0.8161, 42.3503) (-0.8181, 42.3407) (-0.8201, 42.3311) (-0.8221, 42.3215) (-0.824, 42.312) (-0.8259, 42.3025) (-0.8279, 42.293) (-0.8297, 42.2836) (-0.8316, 42.2742) (-0.8334, 42.2649) (-0.8353, 42.2556) (-0.8371, 42.2464) (-0.8388, 42.2372) (-0.8406, 42.228) (-0.8423, 42.2189) (-0.844, 42.2098) (-0.8457, 42.2008) (-0.8474, 42.1918) (-0.849, 42.1828) (-0.8507, 42.1739) (-0.8523, 42.1651) (-0.8538, 42.1563) (-0.8554, 42.1475) (-0.8569, 42.1388) (-0.8585, 42.1301) (-0.86, 42.1214) (-0.8614, 42.1128) (-0.8629, 42.1043) (-0.8643, 42.0958) (-0.8657, 42.0873) (-0.8671, 42.0789) (-0.8685, 42.0706) (-0.8698, 42.0623) (-0.8712, 42.054) (-0.8725, 42.0458) (-0.8738, 42.0376) (-0.875, 42.0295) (-0.8763, 42.0214) (-0.8775, 42.0134) (-0.8787, 42.0054) (-0.8799, 41.9975) (-0.8811, 41.9896) (-0.8822, 41.9818) (-0.8834, 41.974) (-0.8845, 41.9663) (-0.8856, 41.9586) (-0.8866, 41.951) (-0.8877, 41.9434) (-0.8887, 41.9359) (-0.8897, 41.9284) (-0.8907, 41.921) (-0.8917, 41.9137) (-0.8927, 41.9063) (-0.8936, 41.8991) (-0.8945, 41.8919) (-0.8954, 41.8847) (-0.8963, 41.8777) (-0.8972, 41.8706) (-0.898, 41.8636) (-0.8989, 41.8567) (-0.8997, 41.8498) (-0.9005, 41.843) (-0.9012, 41.8363) (-0.902, 41.8296) (-0.9027, 41.823) (-0.9035, 41.8164) (-0.9042, 41.8099) (-0.9049, 41.8034) (-0.9055, 41.797) (-0.9062, 41.7906) (-0.9068, 41.7844) (-0.9075, 41.7781) (-0.9081, 41.772) (-0.9087, 41.7659) (-0.9092, 41.7599) (-0.9098, 41.7539) (-0.9103, 41.748) (-0.9109, 41.7421) (-0.9114, 41.7363) (-0.9119, 41.7306) (-0.9124, 41.725) (-0.9128, 41.7194) (-0.9133, 41.7139) (-0.9137, 41.7084) (-0.9141, 41.703) (-0.9146, 41.6977) (-0.915, 41.6925) (-0.9153, 41.6873) (-0.9157, 41.6822) (-0.9161, 41.6771) (-0.9164, 41.6722) (-0.9167, 41.6673) (-0.917, 41.6624) (-0.9173, 41.6577) (-0.9176, 41.653) (-0.9179, 41.6484) (-0.9182, 41.6439) (-0.9184, 41.6394) (-0.9186, 41.635) (-0.9189, 41.6307) (-0.9191, 41.6265) (-0.9193, 41.6223) (-0.9195, 41.6183) (-0.9197, 41.6143) (-0.9198, 41.6103) (-0.92, 41.6065) (-0.9201, 41.6028) (-0.9203, 41.5991) (-0.9204, 41.5955) (-0.9205, 41.592) (-0.9206, 41.5886) (-0.9208, 41.5852) (-0.9208, 41.582) (-0.9209, 41.5788) (-0.921, 41.5758) (-0.9211, 41.5728) (-0.9211, 41.5699) (-0.9212, 41.5671) (-0.9212, 41.5644) (-0.9213, 41.5618) (-0.9213, 41.5592) (-0.9214, 41.5568) (-0.9214, 41.5545) (-0.9214, 41.5522) (-0.9214, 41.5501) (-0.9214, 41.5481) (-0.9214, 41.5461) (-0.9214, 41.5443) (-0.9214, 41.5425) (-0.9214, 41.5409) (-0.9214, 41.5394) (-0.9214, 41.538) (-0.9214, 41.5367) (-0.9214, 41.5355) (-0.9214, 41.5344) (-0.9213, 41.5334) (-0.9213, 41.5325) (-0.9213, 41.5318) (-0.9213, 41.5313) (-0.9213, 41.5309) (-0.9213, 41.5307) (-0.9213, 41.5307) knots -1 -1 -1 -1 -1 -1 -0.99583333 -0.99166667 -0.9875 -0.98333333 -0.97916667 -0.975 -0.97083333 -0.96666667 -0.9625 -0.95833333 -0.95416667 -0.95 -0.94583333 -0.94166667 -0.9375 -0.93333333 -0.92916667 -0.925 -0.92083333 -0.91666667 -0.9125 -0.90833333 -0.90416667 -0.9 -0.89583333 -0.89166667 -0.8875 -0.88333333 -0.87916667 -0.875 -0.87083333 -0.86666667 -0.8625 -0.85833333 -0.85416667 -0.85 -0.84583333 -0.84166667 -0.8375 -0.83333333 -0.82916667 -0.825 -0.82083333 -0.81666667 -0.8125 -0.80833333 -0.80416667 -0.8 -0.79583333 -0.79166667 -0.7875 -0.78333333 -0.77916667 -0.775 -0.77083333 -0.76666667 -0.7625 -0.75833333 -0.75416667 -0.75 -0.74583333 -0.74166667 -0.7375 -0.73333333 -0.72916667 -0.725 -0.72083333 -0.71666667 -0.7125 -0.70833333 -0.70416667 -0.7 -0.69583333 -0.69166667 -0.6875 -0.68333333 -0.67916667 -0.675 -0.67083333 -0.66666667 -0.6625 -0.65833333 -0.65416667 -0.65 -0.64583333 -0.64166667 -0.6375 -0.63333333 -0.62916667 -0.625 -0.62083333 -0.61666667 -0.6125 -0.60833333 -0.60416667 -0.6 -0.59583333 -0.59166667 -0.5875 -0.58333333 -0.57916667 -0.575 -0.57083333 -0.56666667 -0.5625 -0.55833333 -0.55416667 -0.55 -0.54583333 -0.54166667 -0.5375 -0.53333333 -0.52916667 -0.525 -0.52083333 -0.51666667 -0.5125 -0.50833333 -0.50416667 -0.5 -0.49583333 -0.49166667 -0.4875 -0.48333333 -0.47916667 -0.475 -0.47083333 -0.46666667 -0.4625 -0.45833333 -0.45416667 -0.45 -0.44583333 -0.44166667 -0.4375 -0.43333333 -0.42916667 -0.425 -0.42083333 -0.41666667 -0.4125 -0.40833333 -0.40416667 -0.4 -0.39583333 -0.39166667 -0.3875 -0.38333333 -0.37916667 -0.375 -0.37083333 -0.36666667 -0.3625 -0.35833333 -0.35416667 -0.35 -0.34583333 -0.34166667 -0.3375 -0.33333333 -0.32916667 -0.325 -0.32083333 -0.31666667 -0.3125 -0.30833333 -0.30416667 -0.3 -0.29583333 -0.29166667 -0.2875 -0.28333333 -0.27916667 -0.275 -0.27083333 -0.26666667 -0.2625 -0.25833333 -0.25416667 -0.25 -0.24583333 -0.24166667 -0.2375 -0.23333333 -0.22916667 -0.225 -0.22083333 -0.21666667 -0.2125 -0.20833333 -0.20416667 -0.2 -0.19583333 -0.19166667 -0.1875 -0.18333333 -0.17916667 -0.175 -0.17083333 -0.16666667 -0.1625 -0.15833333 -0.15416667 -0.15 -0.14583333 -0.14166667 -0.1375 -0.13333333 -0.12916667 -0.125 -0.12083333 -0.11666667 -0.1125 -0.10833333 -0.10416667 -0.1 -0.09583333 -0.09166667 -0.0875 -0.08333333 -0.07916667 -0.075 -0.07083333 -0.06666667 -0.0625 -0.05833333 -0.05416667 -0.05 -0.04583333 -0.04166667 -0.0375 -0.03333333 -0.02916667 -0.025 -0.02083333 -0.01666667 -0.0125 -0.00833333 -0.00416667 0 0 0 0 0 0
  arc A55 (-12.1618, 41.0147) -> (-13.0527, 40.6181) centre (0, 12.5) ccw
  line L113 (-15.3132, 37.1806) -> (-15.3128, 37.1799)
  line L114 (-3.9507, 41.2745) -> (-3.9106, 40.9828)
  arc A56 (-12.5209, 38.3803) -> (-13.578, 37.8417) centre (0, 12.5) ccw
  line L115 (-20.9569, 32.6094) -> (-20.9575, 32.61)
  arc A57 (-22.7084, 33.6029) -> (-23.3609, 32.8781) centre (0, 12.5) ccw
  arc A58 (-19.9055, 33.2445) -> (-20.7445, 32.4055) centre (0, 12.5) ccw
  arc A59 (-20.3781, 35.8609) -> (-21.1029, 35.2084) centre (0, 12.5) ccw
  arc A60 (-17.8246, 37.863) -> (-18.6136, 37.2898) centre (0, 12.5) ccw
  arc A61 (-17.6281, 35.2115) -> (-18.5501, 34.4649) centre (0, 12.5) ccw
  line L116 (-8.0945, 40.3937) -> (-8.0948, 40.3945)
  arc A62 (-6.8665, 40.418) -> (-8.0125, 40.1109) centre (0, 12.5) ccw
  line L117 (-9.8469, 39.8243) -> (-9.7471, 39.5473)
  spline S45 degree 5 poles (-6.9214, 42.7174) (-6.9218, 42.7148) (-6.9225, 42.7094) (-6.9236, 42.7014) (-6.925, 42.6907) (-6.9267, 42.6773) (-6.9284, 42.664) (-6.9301, 42.6507) (-6.9317, 42.6375) (-6.9334, 42.6242) (-6.935, 42.611) (-6.9366, 42.5979) (-6.9382, 42.5847) (-6.9398, 42.5716) (-6.9413, 42.5585) (-6.9428, 42.5455) (-6.9443, 42.5324) (-6.9458, 42.5194) (-6.9473, 42.5065) (-6.9487, 42.4935) (-6.9501, 42.4806) (-6.9516, 42.4678) (-6.9529, 42.4549) (-6.9543, 42.4421) (-6.9556, 42.4293) (-6.957, 42.4166) (-6.9583, 42.4039) (-6.9596, 42.3912) (-6.9608, 42.3785) (-6.9621, 42.3659) (-6.9633, 42.3533) (-6.9645, 42.3407) (-6.9657, 42.3282) (-6.9669, 42.3157) (-6.968, 42.3032) (-6.9691, 42.2908) (-6.9702, 42.2784) (-6.9713, 42.266) (-6.9724, 42.2537) (-6.9735, 42.2414) (-6.9745, 42.2291) (-6.9755, 42.2169) (-6.9765, 42.2047) (-6.9775, 42.1925) (-6.9784, 42.1803) (-6.9794, 42.1682) (-6.9803, 42.1562) (-6.9812, 42.1441) (-6.9821, 42.1321) (-6.983, 42.1201) (-6.9838, 42.1082) (-6.9846, 42.0963) (-6.9855, 42.0844) (-6.9863, 42.0726) (-6.987, 42.0608) (-6.9878, 42.049) (-6.9885, 42.0373) (-6.9892, 42.0256) (-6.99, 42.014) (-6.9906, 42.0023) (-6.9913, 41.9907) (-6.992, 41.9792) (-6.9926, 41.9677) (-6.9932, 41.9562) (-6.9938, 41.9447) (-6.9944, 41.9333) (-6.995, 41.922) (-6.9955, 41.9106) (-6.996, 41.8993) (-6.9965, 41.8881) (-6.997, 41.8768) (-6.9975, 41.8657) (-6.998, 41.8545) (-6.9984, 41.8434) (-6.9989, 41.8323) (-6.9993, 41.8213) (-6.9997, 41.8103) (-7.0001, 41.7993) (-7.0004, 41.7884) (-7.0008, 41.7775) (-7.0011, 41.7667) (-7.0014, 41.7559) (-7.0017, 41.7451) (-7.002, 41.7344) (-7.0023, 41.7237) (-7.0025, 41.713) (-7.0028, 41.7024) (-7.003, 41.6919) (-7.0032, 41.6813) (-7.0034, 41.6708) (-7.0035, 41.6604) (-7.0037, 41.65) (-7.0038, 41.6396) (-7.004, 41.6293) (-7.0041, 41.619) (-7.0042, 41.6088) (-7.0043, 41.5986) (-7.0043, 41.5884) (-7.0044, 41.5783) (-7.0044, 41.5682) (-7.0045, 41.5582) (-7.0045, 41.5482) (-7.0045, 41.5383) (-7.0045, 41.5284) (-7.0044, 41.5185) (-7.0044, 41.5087) (-7.0043, 41.4989) (-7.0043, 41.4892) (-7.0042, 41.4795) (-7.0041, 41.4698) (-7.004, 41.4602) (-7.0038, 41.4507) (-7.0037, 41.4412) (-7.0036, 41.4317) (-7.0034, 41.4223) (-7.0032, 41.4129) (-7.003, 41.4036) (-7.0028, 41.3943) (-7.0026, 41.3851) (-7.0024, 41.3759) (-7.0021, 41.3668) (-7.0019, 41.3577) (-7.0016, 41.3486) (-7.0014, 41.3396) (-7.0011, 41.3307) (-7.0008, 41.3218) (-7.0005, 41.3129) (-7.0001, 41.3041) (-6.9998, 41.2953) (-6.9995, 41.2866) (-6.9991, 41.278) (-6.9987, 41.2694) (-6.9984, 41.2608) (-6.998, 41.2523) (-6.9976, 41.2438) (-6.9972, 41.2354) (-6.9968, 41.227) (-6.9963, 41.2187) (-6.9959, 41.2105) (-6.9954, 41.2023) (-6.995, 41.1941) (-6.9945, 41.186) (-6.994, 41.178) (-6.9936, 41.17) (-6.9931, 41.162) (-6.9926, 41.1541) (-6.9921, 41.1463) (-6.9915, 41.1385) (-6.991, 41.1307) (-6.9905, 41.1231) (-6.9899, 41.1154) (-6.9894, 41.1079) (-6.9888, 41.1004) (-6.9882, 41.0929) (-6.9877, 41.0855) (-6.9871, 41.0781) (-6.9865, 41.0709) (-6.9859, 41.0636) (-6.9853, 41.0564) (-6.9847, 41.0493) (-6.9841, 41.0423) (-6.9835, 41.0353) (-6.9828, 41.0283) (-6.9822, 41.0214) (-6.9816, 41.0146) (-6.9809, 41.0078) (-6.9803, 41.0011) (-6.9796, 40.9945) (-6.9789, 40.9879) (-6.9783, 40.9814) (-6.9776, 40.9749) (-6.9769, 40.9685) (-6.9763, 40.9622) (-6.9756, 40.9559) (-6.9749, 40.9497) (-6.9742, 40.9435) (-6.9735, 40.9374) (-6.9728, 40.9314) (-6.9721, 40.9255) (-6.9714, 40.9196) (-6.9707, 40.9137) (-6.97, 40.908) (-6.9693, 40.9023) (-6.9686, 40.8966) (-6.9679, 40.8911) (-6.9672, 40.8856) (-6.9665, 40.8802) (-6.9658, 40.8748) (-6.9651, 40.8695) (-6.9644, 40.8643) (-6.9637, 40.8592) (-6.963, 40.8541) (-6.9623, 40.8491) (-6.9616, 40.8442) (-6.9609, 40.8393) (-6.9602, 40.8345) (-6.9595, 40.8298) (-6.9588, 40.8252) (-6.9581, 40.8206) (-6.9574, 40.8161) (-6.9568, 40.8117) (-6.9561, 40.8074) (-6.9554, 40.8031) (-6.9547, 40.7989) (-6.9541, 40.7948) (-6.9534, 40.7908) (-6.9528, 40.7868) (-6.9521, 40.783) (-6.9515, 40.7792) (-6.9508, 40.7755) (-6.9502, 40.7719) (-6.9496, 40.7683) (-6.949, 40.7649) (-6.9484, 40.7615) (-6.9478, 40.7582) (-6.9472, 40.755) (-6.9466, 40.7519) (-6.9461, 40.7489) (-6.9455, 40.746) (-6.945, 40.7431) (-6.9445, 40.7404) (-6.9439, 40.7377) (-6.9434, 40.7351) (-6.9429, 40.7327) (-6.9425, 40.7303) (-6.942, 40.728) (-6.9416, 40.7258) (-6.9411, 40.7237) (-6.9407, 40.7217) (-6.9403, 40.7198) (-6.9399, 40.718) (-6.9396, 40.7163) (-6.9392, 40.7147) (-6.9389, 40.7132) (-6.9386, 40.7118) (-6.9383, 40.7106) (-6.9381, 40.7094) (-6.9378, 40.7083) (-6.9376, 40.7074) (-6.9374, 40.7065) (-6.9372, 40.7058) (-6.9371, 40.7053) (-6.937, 40.705) (-6.937, 40.7048) (-6.937, 40.7047) knots -1 -1 -1 -1 -1 -1 -0.99583333 -0.99166667 -0.9875 -0.98333333 -0.97916667 -0.975 -0.97083333 -0.96666667 -0.9625 -0.95833333 -0.95416667 -0.95 -0.94583333 -0.94166667 -0.9375 -0.93333333 -0.92916667 -0.925 -0.92083333 -0.91666667 -0.9125 -0.90833333 -0.90416667 -0.9 -0.89583333 -0.89166667 -0.8875 -0.88333333 -0.87916667 -0.875 -0.87083333 -0.86666667 -0.8625 -0.85833333 -0.85416667 -0.85 -0.84583333 -0.84166667 -0.8375 -0.83333333 -0.82916667 -0.825 -0.82083333 -0.81666667 -0.8125 -0.80833333 -0.80416667 -0.8 -0.79583333 -0.79166667 -0.7875 -0.78333333 -0.77916667 -0.775 -0.77083333 -0.76666667 -0.7625 -0.75833333 -0.75416667 -0.75 -0.74583333 -0.74166667 -0.7375 -0.73333333 -0.72916667 -0.725 -0.72083333 -0.71666667 -0.7125 -0.70833333 -0.70416667 -0.7 -0.69583333 -0.69166667 -0.6875 -0.68333333 -0.67916667 -0.675 -0.67083333 -0.66666667 -0.6625 -0.65833333 -0.65416667 -0.65 -0.64583333 -0.64166667 -0.6375 -0.63333333 -0.62916667 -0.625 -0.62083333 -0.61666667 -0.6125 -0.60833333 -0.60416667 -0.6 -0.59583333 -0.59166667 -0.5875 -0.58333333 -0.57916667 -0.575 -0.57083333 -0.56666667 -0.5625 -0.55833333 -0.55416667 -0.55 -0.54583333 -0.54166667 -0.5375 -0.53333333 -0.52916667 -0.525 -0.52083333 -0.51666667 -0.5125 -0.50833333 -0.50416667 -0.5 -0.49583333 -0.49166667 -0.4875 -0.48333333 -0.47916667 -0.475 -0.47083333 -0.46666667 -0.4625 -0.45833333 -0.45416667 -0.45 -0.44583333 -0.44166667 -0.4375 -0.43333333 -0.42916667 -0.425 -0.42083333 -0.41666667 -0.4125 -0.40833333 -0.40416667 -0.4 -0.39583333 -0.39166667 -0.3875 -0.38333333 -0.37916667 -0.375 -0.37083333 -0.36666667 -0.3625 -0.35833333 -0.35416667 -0.35 -0.34583333 -0.34166667 -0.3375 -0.33333333 -0.32916667 -0.325 -0.32083333 -0.31666667 -0.3125 -0.30833333 -0.30416667 -0.3 -0.29583333 -0.29166667 -0.2875 -0.28333333 -0.27916667 -0.275 -0.27083333 -0.26666667 -0.2625 -0.25833333 -0.25416667 -0.25 -0.24583333 -0.24166667 -0.2375 -0.23333333 -0.22916667 -0.225 -0.22083333 -0.21666667 -0.2125 -0.20833333 -0.20416667 -0.2 -0.19583333 -0.19166667 -0.1875 -0.18333333 -0.17916667 -0.175 -0.17083333 -0.16666667 -0.1625 -0.15833333 -0.15416667 -0.15 -0.14583333 -0.14166667 -0.1375 -0.13333333 -0.12916667 -0.125 -0.12083333 -0.11666667 -0.1125 -0.10833333 -0.10416667 -0.1 -0.09583333 -0.09166667 -0.0875 -0.08333333 -0.07916667 -0.075 -0.07083333 -0.06666667 -0.0625 -0.05833333 -0.05416667 -0.05 -0.04583333 -0.04166667 -0.0375 -0.03333333 -0.02916667 -0.025 -0.02083333 -0.01666667 -0.0125 -0.00833333 -0.00416667 0 0 0 0 0 0